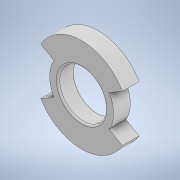
# Autodesk Inventor part: soporte bomba
Saved by Autodesk Inventor 2021 (Build 250183000, 183)
## iProperties
Created: 2020-11-18
Part Number: soporte bomba
Material: Generic
Document SubType Name: Modeling
Designer: Miguel
Density: 1 g/cm^3
Appearance: Default
Author: Miguel
Autodesk Inventor part; units mm, degrees
ref_plane "YZ Plane" through (0, 0, 0) normal (1, 0, 0) x (0, 1, 0)
ref_plane "XZ Plane" through (0, 0, 0) normal (0, 1, 0) x (-1, 0, 0)
ref_plane "XY Plane" through (0, 0, 0) normal (0, 0, 1) x (1, 0, 0)
sketch "Sketch1" plane through (0, 0, 0) normal (0, 0, 1) x (1, 0, 0)
  circle A0 centre (0, 0) radius 28
  circle A1 centre (0, 0) radius 14
  circle A2 centre (0, 0) radius 19
  line L0 (0, 0) -> (-24.2487, 14)
  line L1 (0, 0) -> (24.2487, 14)
  line L2 (0, 0) -> (6.8345, 0)
  line L3 (0, 0) -> (24.2487, -14)
  line L4 (0, 0) -> (-24.2487, -14)
  point P0 (-16.4545, 9.5)
  point P1 (16.4545, 9.5)
  point P2 (-16.4545, -9.5)
  point P3 (16.4545, -9.5)
  dimension "d0" = 56
  dimension "d1" = 28
  dimension "d2" = 5
  dimension "d3" = 120
  dimension "d4" = 30
  dimension "d8" = 120
  dimension "d9" = 60
  constraints: 10 end point, 4 point on circle, 3 centre point, 3 coincident, 1 horizontal
  measures "d0" diameter of A0
  measures "d1" diameter of A1
  measures "d2" radial gap between concentric circles of A2 A1
  measures "d3" angle of L1 L0
  measures "d4" angle of L1 L2
  measures "d8" angle of L3 L4
  measures "d9" angle of L1 L3
extrude "Extrusion1" add sketch "Sketch1" along normal blind 10 contours L1 A2 L0 A0 | L1 A1 L0 A2 | A2 L3 A1 L1 | A2 L4 A1 L3 | L0 A1 L4 A2
fillet "Fillet1" radius 1 2 edges at (-14, 0, 0) (-14, 0, 10)
extrude "Extrusion2" add sketch "Sketch1" along normal blind 10 contours A0 L4 A2 L3
body "Solid1"
